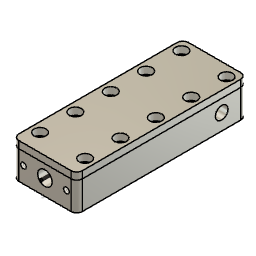
pulse pick-off v3 (Autodesk Fusion 360 design; units mm, degrees)
Autodesk Fusion 360 part; units mm, degrees
note: some values were not read from the file. Chosen so that the rebuilt part matches the saved one: which pieces of a blend or face edit are solid. Set by a fixed rule: the direction of a hole.
sketch "Sketch1" plane through (0, 0, 0) normal (0, 1, 0) x (1, 0, 0)
  line L0 (-9, 24) -> (9, 24)
  line L1 (9, 24) -> (9, -24)
  line L2 (9, -24) -> (-9, -24)
  line L3 (-9, -24) -> (-9, 24)
  line L4 (-3.75, -20) -> (-3.75, 20)
  line L5 (-3.75, 20) -> (3.75, 20)
  line L6 (3.75, 20) -> (3.75, -20)
  line L7 (0, 24) -> (0, -24) construction
  line L8 (-3.75, -20) -> (3.75, -20)
  line L9 (-3.75, 15) -> (-2.5, 15)
  line L10 (-2.5, 15) -> (-2.5, 20)
  line L11 (2.5, 20) -> (2.5, 15)
  line L12 (2.5, 15) -> (3.75, 15)
  line L13 (-6.375, 24) -> (-6.375, -24) construction
  point P0 (-6.375, 21)
  point P1 (-6.375, 11)
  point P2 (-6.375, 1)
  point P3 (-6.375, -9)
  point P4 (-6.375, -19)
  point P5 (6.375, 21)
  point P6 (6.375, 11)
  point P7 (6.375, 1)
  point P8 (6.375, -9)
  point P9 (6.375, -19)
  dimension "d2" = 18
  dimension "d3" = 4
  dimension "d4" = 7.5
  dimension "d5" = 4
  dimension "d6" = 5
  dimension "d7" = 35
  dimension "d8" = 5
  dimension "d11" = 40
  dimension "d12" = 0
  dimension "d13" = 3
  dimension "d14" = 5
  constraint horizontal L0
  constraint perpendicular L0 L1
  constraint parallel L0 L2
  constraint parallel L1 L3
  constraint perpendicular L4 L5
  constraint midpoint L0 L7.start
  constraint midpoint L2 L7.end
  constraint midpoint origin L7
  constraint symmetric L4 L6 L7
  constraint perpendicular L6 L8
  constraint coincident L4 L9.start
  constraint perpendicular L4 L9
  constraint coincident L5 L10.end
  constraint perpendicular L5 L10
  constraint coincident L5 L11.start
  constraint perpendicular L5 L11
  constraint coincident L6 L12.end
  constraint perpendicular L6 L12
  constraint collinear L9 L12
  constraint coincident L0 L13.start
  constraint coincident L2 L13.end
  constraint perpendicular L2 L13
  constraint coincident L13 P0
  constraint symmetric L7 P0 P5
  constraint symmetric L7 P1 P6
  constraint symmetric L7 P2 P7
  constraint symmetric L7 P3 P8
  constraint symmetric L7 P4 P9
  measures "d2" distance of L0.start L0.end
  measures "d3" distance of L0 L5
  measures "d4" distance of L4 L6
  measures "d5" distance of L2 L8
  measures "d6" distance of L10 L11
  measures "d7" distance of L8 L9
  measures "d8" distance of L5 L9
  measures "d13" distance of L0 P0
  measures "d14" distance of L2 P4
extrude "Extrude1" add sketch "Sketch1" against normal blind 8 contours L0 L1 L2 L3 | L4 L5 L6 L8 L9 L10 L11 L12 | L4 L5 L9 L10 | L5 L6 L11 L12 makes body 1
extrude "Extrude2" cut sketch "Sketch1" against normal blind 7 contours L4 L5 L6 L8 L9 L10 L11 L12 bodies 1
sketch "Sketch2" plane through (9, 0, 0) normal (1, 0, 0) x (0, 0, -1)
  line L0 (24, 0) -> (-24, 0)
  line L1 (-24, 0) -> (-24, -8)
  line L2 (-24, -8) -> (24, -8)
  line L3 (24, -8) -> (24, 0)
  line L4 (24, 0) -> (-24, 0)
  point P0 (17, -3.5)
  dimension "d20" = 3.5
  dimension "d21" = 7
  measures "d20" distance of P0 L4
  measures "d21" distance of L3 P0
hole "Hole1" at (9, -3.5, -17) direction (-1, 0, 0) diameter 3.6 end through all bodies 1
sketch "Sketch3" plane through (0, 0, 24) normal (0, 0, 1) x (1, 0, 0)
  line L0 (9, 0) -> (-9, 0)
  line L1 (-9, 0) -> (-9, -8)
  line L2 (-9, -8) -> (9, -8)
  line L3 (9, -8) -> (9, 0)
  line L4 (-6.075, -3.5) -> (6.075, -3.5) construction
  point P0 (0, -3.5)
  dimension "d25" = 3.5
  dimension "d48" = 12.15
  constraint vertical origin P0
  constraint horizontal L4
  constraint midpoint P0 L4
  measures "d25" distance of origin P0
  measures "d48" distance of L4.start L4.end
hole "Hole2" at (0, -3.5, 24) direction (0, 0, -1) diameter 4.1 depth 20 tip angle 118 bodies 1
extrude "Extrude3" add sketch "Sketch1" along normal blind 2 separate body contours L0 L1 L2 L3 | L4 L5 L6 L8 L9 L10 L11 L12 | L4 L5 L9 L10 | L5 L6 L11 L12 makes body 2
fillet "Fillet1" radius 1.6 16 edges at (-3.75, -3.5, 20) (3.75, -3.5, 20) (-3.75, -3.5, -15) (-2.5, -3.5, -15) (-2.5, -3.5, -20) (2.5, -3.5, -20) (2.5, -3.5, -15) (3.75, -3.5, -15) (9, -4, 24) (-9, -4, 24) (-9, -4, -24) (9, -4, -24) (9, 1, 24) (-9, 1, 24) (-9, 1, -24) (9, 1, -24) on bodies 1 2
cylinder "CylinderPrimitive1" add diameter 7 height 27 placed x (1, 0, 0) y (0, 0, -1) z (0, 1, 0) at (0, 0, 0) separate body makes body 3
cylinder "CylinderPrimitive2" add diameter 0.8 height 10 placed x (1, 0, 0) y (0, 0, -1) z (0, 1, 0) at (0, 27, 0) bodies 3
cylinder "CylinderPrimitive3" add diameter 0.8 height 10 placed x (1, 0, 0) y (0, 0, 1) z (0, -1, 0) at (0, 0, 0) bodies 3
hole "Hole3" at (-6.375, 0, 19) at (-6.375, 0, 9) at (-6.375, 0, -1) at (-6.375, 0, -11) at (-6.375, 0, -21) at (6.375, 0, -21) at (6.375, 0, -11) at (6.375, 0, -1) at (6.375, 0, 9) at (6.375, 0, 19) direction (0, -1, 0) diameter 2.529 depth 20 tip angle 118 bodies 1
thread "Thread1" "ISO Metric profile 3.0 M3x0.5 6H" thread offset 0 thread depth 10
hole "Hole4" at (-6.375, 0, -21) at (-6.375, 0, -11) at (-6.375, 0, -1) at (-6.375, 0, 9) at (-6.375, 0, 19) at (6.375, 0, 19) at (6.375, 0, 9) at (6.375, 0, -1) at (6.375, 0, -11) at (6.375, 0, -21) direction (0, 1, 0) diameter 3.4 depth 20 tip angle 118 bodies 2
hole "Hole5" at (-6.075, -3.5, 24) at (6.075, -3.5, 24) direction (0, 0, -1) diameter 1.623 depth 5 tip angle 118 bodies 1
thread "Thread2" "ISO Metric profile 2.0 M2x0.4 6H" thread offset 0 thread depth 10
copy_body "Body->Comp1" bodies 1 removing the originals makes body 4 in component "case"
copy_body "Body->Comp2" bodies 2 removing the originals makes body 5 in component "lid"
copy_body "Body->Comp3" bodies 3 removing the originals makes body 6 in component "resistor"
component "case" placed x (1, 0, 0) y (0, 1, 0) z (0, 0, 1) at (0, 0, 0)
component "lid" placed x (1, 0, 0) y (0, 1, 0) z (0, 0, 1) at (0, 0, 0)
component "resistor" placed x (1, 0, 0) y (0, 0, 1) z (0, -1, 0) at (0, -3.5, -12)
named bodies: "case", "lid", "resistor"
